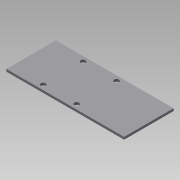
# Autodesk Inventor part: 13_Zwischenebene_LCD
Saved by Autodesk Inventor 2015 (Build 190159000, 159)
## iProperties
Created: 2016-03-06
Part Number: 13_Zwischenebene_LCD
Material: Generisch
Document SubType Name: Modeling
Designer: Bene
Density: 1 g/cm^3
Appearance: Vorgabe
Author: Bene
Autodesk Inventor part; units mm, degrees
ref_plane "YZ Plane" through (0, 0, 0) normal (1, 0, 0) x (0, 1, 0)
ref_plane "XZ Plane" through (0, 0, 0) normal (0, 1, 0) x (-1, 0, 0)
ref_plane "XY Plane" through (0, 0, 0) normal (0, 0, 1) x (1, 0, 0)
sketch "Skizze1" plane through (0, 0, 0) normal (0, 0, 1) x (1, 0, 0)
  arc A0 (-10.0563, 3.3011) -> (-12.2178, -3.2473) centre (-1.2178, -3.2473) ccw projected
  line L0 (-12.2178, -3.2473) -> (9.7822, -3.2473) projected
  arc A1 (9.7822, -3.2473) -> (7.6207, 3.3011) centre (-1.2178, -3.2473) ccw projected
  arc A2 (-3.7041, 1.8719) -> (7.6207, 3.3011) centre (-1.2178, 27.7527) ccw projected
  line L1 (-3.7041, 1.8719) -> (-4.2446, 1.7527) projected
  line L2 (-4.2446, 1.7527) -> (-4.7816, 1.7527) projected
  line L3 (-4.7816, 1.7527) -> (-6.4898, 2.2928) projected
  arc A3 (-10.0563, 3.3011) -> (-6.4898, 2.2928) centre (-1.2178, 27.7527) ccw projected
  arc A4 (-12.2178, 58.7527) -> (-10.0563, 52.2043) centre (-1.2178, 58.7527) ccw projected
  arc A5 (7.6207, 52.2043) -> (-10.0563, 52.2043) centre (-1.2178, 27.7527) ccw projected
  arc A6 (7.6207, 52.2043) -> (9.7822, 58.7527) centre (-1.2178, 58.7527) ccw projected
  line L4 (9.7822, 58.7527) -> (-12.2178, 58.7527) projected
  line L5 (85.2075, 58.7527) -> (80.2075, 58.7527) projected
  line L6 (80.2075, 58.7527) -> (80.2075, 53.7527) projected
  line L7 (80.2075, 53.7527) -> (85.2075, 53.7527) projected
  line L8 (85.2075, 53.7527) -> (85.2075, 58.7527) projected
  line L9 (85.2075, -3.2473) -> (85.2075, 1.7527) projected
  line L10 (85.2075, 1.7527) -> (80.2075, 1.7527) projected
  line L11 (80.2075, 1.7527) -> (80.2075, -3.2473) projected
  line L12 (80.2075, -3.2473) -> (85.2075, -3.2473) projected
  circle A7 centre (19.8794, 52.7527) radius 3 projected
  circle A8 centre (19.8794, 2.7527) radius 3 projected
  circle A9 centre (-22.1206, 2.7527) radius 3 projected
  circle A10 centre (-22.1206, 52.7527) radius 3 projected
  line L13 (85.2075, 58.7527) -> (-62.1847, 58.7527)
  line L14 (-62.1847, 58.7527) -> (-62.1847, -3.2473)
  line L15 (-62.1847, -3.2473) -> (85.2075, -3.2473)
  line L16 (85.2075, -3.2473) -> (85.2075, 58.7527)
  point P0 (0, 0)
  constraints: 8 end point, 2 parallel, 1 horizontal, 1 perpendicular
extrude "Extrusion1" add sketch "Skizze1" along normal blind 3
sketch "Skizze2" plane through (0, 0, 3) normal (0, 0, 1) x (1, 0, 0)
  circle A0 centre (-3.1206, 27.7527) radius 15 projected
  line L0 (85.2075, 58.7527) -> (-62.1847, 58.7527) projected
  line L1 (-62.1847, -3.2473) -> (85.2075, -3.2473) projected
  line L2 (27.3951, 58.7527) -> (31.3951, 58.7527)
  line L3 (31.3951, 58.7527) -> (31.3951, -3.2473)
  line L4 (31.3951, -3.2473) -> (27.3951, -3.2473)
  line L5 (27.3951, -3.2473) -> (27.3951, 58.7527)
  line L6 (35.5129, 58.7527) -> (39.5129, 58.7527)
  line L7 (39.5129, 58.7527) -> (39.5129, 3.8427)
  line L8 (39.5129, 3.8427) -> (35.5129, 3.8427)
  line L9 (35.5129, 3.8427) -> (35.5129, 58.7527)
  line L10 (85.2075, -3.2473) -> (85.2075, 58.7527) projected
  line L11 (39.5129, 3.8427) -> (85.2075, 3.8427)
  line L12 (85.2075, 3.8427) -> (85.2075, 7.8427)
  line L13 (85.2075, 7.8427) -> (39.5129, 7.8427)
  line L14 (39.5129, 7.8427) -> (39.5129, 3.8427)
  point P0 (0, 0)
  dimension "d2" = 4
  dimension "d3" = 4
  dimension "d4" = 45.6946
  dimension "d5" = 4
  constraints: 24 end point, 6 parallel, 4 point on line, 3 horizontal, 3 perpendicular
  measures "d2" distance of L3.end L4.end
  measures "d3" distance of L7.end L8.end
  measures "d4" distance of L13.end L12.end
  measures "d5" distance of L12.end L11.end
extrude "Extrusion2" add sketch "Skizze2" along normal blind 35 contours L7 L8 L9 L0 | L10 L11 L7 L13 | L3 L1 L5 L0
sketch "Skizze3" plane through (0, 0, 3) normal (0, 0, 1) x (1, 0, 0)
  line L0 (39.5129, 58.7527) -> (39.5129, 7.8427) projected
  line L1 (39.5129, 7.8427) -> (85.2075, 7.8427) projected
  line L2 (85.2075, 7.8427) -> (85.2075, 58.7527) projected
  line L3 (85.2075, 58.7527) -> (39.5129, 58.7527) projected
  line L4 (27.7822, 53.7527) -> (85.2075, 53.7527) projected
  line L5 (39.5129, 7.8427) -> (85.2075, 7.8427)
  line L6 (85.2075, 7.8427) -> (85.2075, 53.7527)
  line L7 (85.2075, 53.7527) -> (39.5129, 53.7527)
  line L8 (39.5129, 53.7527) -> (39.5129, 7.8427)
  point P0 (0, 0)
  constraints: 8 end point, 2 parallel, 1 horizontal, 1 perpendicular, 1 point on line
extrude "Extrusion3" cut sketch "Skizze3" against normal blind 35 contours L4 L2 L1 L0
sketch "Skizze4" plane through (39.5129, 7.8427, 38) normal (1, 0, 0) x (0, 0, -1)
  line L0 (0, 0) -> (38, 0) projected
  line L1 (38, 45.91) -> (38, 0) projected
  line L2 (35, 45.91) -> (38, 45.91) projected
  line L3 (35, 50.91) -> (35, 45.91) projected
  line L4 (35, 50.91) -> (0, 50.91) projected
  line L5 (0, 0) -> (0, 50.91) projected
  line L6 (0, 0) -> (38, 0) projected
  line L7 (33.1404, 0) -> (3.7306, 0)
  line L8 (3.7306, 0) -> (3.7306, 42.1415)
  line L9 (3.7306, 42.1415) -> (33.1404, 42.1415)
  line L10 (33.1404, 42.1415) -> (33.1404, 0)
  point P0 (38, -7.8427)
  constraints: 8 end point, 2 parallel, 1 horizontal, 1 perpendicular, 1 point on line
extrude "Extrusion4" cut sketch "Skizze4" against normal blind 35 contours L8 L9 L10 L0
